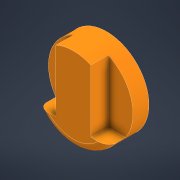
# Autodesk Inventor part: 02_DoF1_Podstawa
Saved by Autodesk Inventor 2022 (Build 260153000, 153)
## iProperties
Created: 2022-05-07
Part Number: 02_DoF1_Podstawa
Material: Generic
Document SubType Name: Modeling
Designer: pzach
Density: 1 g/cm^3
Appearance: Orange
Author: pzach
Autodesk Inventor part; units mm, degrees
ref_plane "YZ Plane" through (0, 0, 0) normal (1, 0, 0) x (0, 1, 0)
ref_plane "XZ Plane" through (0, 0, 0) normal (0, 1, 0) x (-1, 0, 0)
ref_plane "XY Plane" through (0, 0, 0) normal (0, 0, 1) x (1, 0, 0)
sketch "Sketch1" plane through (0, 0, 0) normal (0, 0, 1) x (1, 0, 0)
  circle A0 centre (0, 0) radius 530
  dimension "d0" = 1060
  constraints: 1 centre point, 1 coincident
  measures "d0" diameter of A0
extrude "Extrusion1" add sketch "Sketch1" along normal blind 200
sketch "Sketch2" plane through (0, 0, 200) normal (0, 0, 1) x (1, 0, 0)
  circle A0 centre (0, 0) radius 530 projected
  line L0 (0, 0) -> (0, -300)
  line L1 (-218.4605, -300) -> (-218.4605, 482.882)
  line L2 (436.921, -300) -> (-436.921, -300)
  line L3 (218.4605, -300) -> (218.4605, 482.882)
  point P0 (218.4605, 482.882)
  dimension "d3" = 300
  dimension "d5" = 873.8421
  dimension "d8" = 782.882
  dimension "d9" = 218.4605
  dimension "d10" = 90
  constraints: 8 end point, 3 point on circle, 2 symmetric about line, 1 horizontal, 1 vertical
  measures "d3" distance of L0.start L0.end
  measures "d5" distance of L2.start L2.end
  measures "d8" distance of L1.start L1.end
  measures "d9" distance from line of L1 point (0, 0)
  measures "d10" angle of L2 L1
extrude "Extrusion2" add sketch "Sketch2" along normal blind 218.4605 contours L3 L2 L1 A0 | A0 L2
fillet "Fillet1" radius 100 1 edges at (0, -530, 418.4605)
equation "\"d6\" = d9"
body "Solid1"
